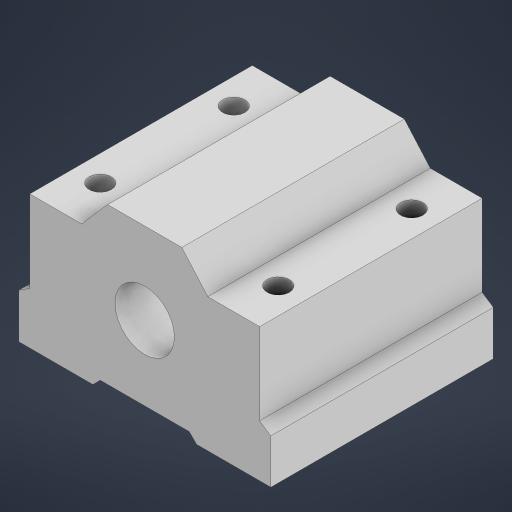
# Autodesk Inventor part: Linear Bearing 8mm Square
Saved by Autodesk Inventor 2024.2 (Build 282272000, 272)
## iProperties
Created: 2024-10-02
Part Number: Linear Bearing 8mm Square
Material: Generic
Document SubType Name: Modeling
Designer: jerem
Density: 1 g/cm^3
Appearance: Default
Author: jerem
Autodesk Inventor part; units mm, degrees
ref_plane "YZ Plane" through (0, 0, 0) normal (1, 0, 0) x (0, 1, 0)
ref_plane "XZ Plane" through (0, 0, 0) normal (0, 1, 0) x (-1, 0, 0)
ref_plane "XY Plane" through (0, 0, 0) normal (0, 0, 1) x (1, 0, 0)
sketch "Sketch1" plane through (0, 0, 0) normal (0, 0, 1) x (1, 0, 0)
  circle A0 centre (0, 0) radius 4
  line L0 (-15.5, 0) -> (-15.5, 7)
  line L1 (-15.5, 7) -> (-8.5, 7)
  line L2 (-8.5, 7) -> (-5, 11)
  line L3 (-5, 11) -> (0, 11)
  line L4 (0, -4) -> (-15.5, -4) construction
  line L5 (-15.5, 0) -> (-15.5, -4)
  line L6 (-17, -11) -> (0, -11) construction
  line L7 (-17, -11) -> (-17, -5)
  line L8 (-17, -5) -> (-15.5, -4)
  line L9 (0, -4) -> (0, -11) construction
  line L10 (0, 4) -> (0, 11) construction
  line L11 (15.5, 0) -> (15.5, 7)
  line L12 (15.5, 7) -> (8.5, 7)
  line L13 (8.5, 7) -> (5, 11)
  line L14 (5, 11) -> (0, 11)
  line L15 (15.5, 0) -> (15.5, -4)
  line L16 (17, -11) -> (17, -5)
  line L17 (17, -5) -> (15.5, -4)
  line L18 (-17, -11) -> (-7, -11)
  line L19 (0, -10) -> (-6, -10)
  line L20 (-7, -11) -> (-6, -10)
  line L21 (17, -11) -> (0, -11) construction
  line L22 (0, -10) -> (6, -10)
  line L23 (7, -11) -> (6, -10)
  line L24 (7, -11) -> (17, -11)
  dimension "d0" = 8
  dimension "d1" = 15.5
  dimension "d2" = 11
  dimension "d3" = 17
  dimension "d4" = 6
  dimension "d5" = 18
  dimension "d6" = 22
  dimension "d7" = 5
  dimension "d8" = 7
  dimension "d19" = 10
  dimension "d20" = 1
  dimension "d21" = 6
  constraints: 52 end point, 9 symmetric about line, 4 vertical, 3 horizontal, 3 point on line, 2 perpendicular, 2 point on circle, 1 centre point, 1 coincident, 1 collinear, 1 line through centre, 1 parallel, 1 tangent
  measures "d0" diameter of A0
  measures "d1" distance from line of L0 point (0, 0)
  measures "d2" distance from line of point (0, 0) L6
  measures "d3" distance of L6.start L6.end
  measures "d4" distance of L6.start L7.end
  measures "d5" distance between parallel lines of L1 L6
  measures "d6" distance between parallel lines of L6 L3
  measures "d7" distance of L2.end L3.end
  measures "d8" distance of L0.end L1.end
  measures "d19" distance of L6.start L18.end
  measures "d20" distance between parallel lines of L6 L19
  measures "d21" distance of L19.start L19.end
extrude "Extrusion1" add sketch "Sketch1" along normal blind 30
sketch "Sketch2" plane through (-15.5, 7, 0) normal (0, 1, 0) x (1, 0, 0)
  circle A0 centre (3.5, -6) radius 1.5
  line L0 (15.5, 0) -> (15.5, -30) construction
  line L1 (32.5, 0) -> (32.5, -30) construction
  line L2 (32.5, -15) -> (-1.5, -15) construction
  line L3 (-1.5, 0) -> (-1.5, -30) construction
  line L4 (27.5, -24) -> (3.5, -24) construction
  line L5 (3.5, -24) -> (3.5, -6) construction
  line L6 (3.5, -6) -> (27.5, -6) construction
  line L7 (27.5, -6) -> (27.5, -24) construction
  line L8 (27.5, -24) -> (3.5, -6) construction
  line L9 (3.5, -24) -> (27.5, -6) construction
  circle A1 centre (27.5, -6) radius 1.5
  circle A2 centre (27.5, -24) radius 1.5
  circle A3 centre (3.5, -24) radius 1.5
  point P0 (15.5, -15)
  dimension "d11" = 3
  dimension "d12" = 24
  dimension "d13" = 18
  dimension "d14" = 3
  dimension "d15" = 3
  dimension "d16" = 3
  constraints: 16 end point, 5 midpoint, 4 centre point, 3 coincident, 2 parallel, 1 horizontal, 1 perpendicular
  measures "d11" diameter of A0
  measures "d12" distance of L5.end L6.end
  measures "d13" distance of L4.end L5.end
  measures "d14" diameter of A3
  measures "d15" diameter of A1
  measures "d16" diameter of A2
extrude "Extrusion2" cut sketch "Sketch2" against normal through all
equation "\"d14\" = d11"
equation "\"d15\" = d11"
equation "\"d16\" = d11"
body "Solid1"
